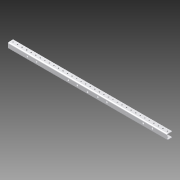
# Autodesk Inventor part: am-0202
Saved by Autodesk Inventor 2012 (Build 160160000, 160)
## iProperties
Category: Chassis
Company: Autodesk Inc.
Created: 2011-12-29
Part Number: am-0202
Document SubType Name: Modeling
Designer: Autodesk Inc.
Density: 1 g/cm^3
Catalog Web Link: http://www.andymark.com/ProductDetails.asp?ProductCode=am%2D0202
Description: C-Channel aluminum piece, for use in the C-Base Drive Chassis.  6 of these items come standard in the C-Base, but only 1 is sh
Vendor: AndyMark
Material: Default
Author: Autodesk Inc.
Autodesk Inventor part; units mm, degrees
ref_plane "YZ Plane" through (0, 0, 0) normal (1, 0, 0) x (0, 1, 0)
ref_plane "XZ Plane" through (0, 0, 0) normal (0, 1, 0) x (-1, 0, 0)
ref_plane "XY Plane" through (0, 0, 0) normal (0, 0, 1) x (1, 0, 0)
sketch "Sketch1" plane through (0, 0, 0) normal (0, 0, 1) x (1, 0, 0)
  line L0 (5.9771, 0) -> (28.2021, 0)
  line L1 (28.2021, 0) -> (28.2021, 3.175)
  line L2 (28.2021, 3.175) -> (5.9771, 3.175)
  line L3 (2.8021, 6.35) -> (2.8021, 25.4)
  line L4 (5.9771, 28.575) -> (28.2021, 28.575)
  line L5 (28.2021, 28.575) -> (28.2021, 31.75)
  line L6 (28.2021, 31.75) -> (5.9771, 31.75)
  line L7 (-0.3729, 25.4) -> (-0.3729, 6.35)
  arc A0 (5.9771, 28.575) -> (2.8021, 25.4) centre (5.9771, 25.4) ccw
  arc A1 (2.8021, 6.35) -> (5.9771, 3.175) centre (5.9771, 6.35) ccw
  arc A2 (5.9771, 31.75) -> (-0.3729, 25.4) centre (5.9771, 25.4) ccw
  arc A3 (-0.3729, 6.35) -> (5.9771, 0) centre (5.9771, 6.35) ccw
  point P0 (0, 0)
  point P1 (-0.3729, 0)
  point P2 (2.8021, 3.175)
  point P3 (2.8021, 28.575)
  dimension "d0" = 28.575
  dimension "d1" = 3.175
  dimension "d2" = 25.4
  dimension "d3" = 25.4
  dimension "d4" = 3.175
  dimension "d5" = 3.175
  dimension "d6" = 6.35
  constraints: 16 end point, 8 point on circle, 8 tangent, 6 point on line, 5 parallel, 4 centre point, 2 equal radius, 1 collinear, 1 horizontal, 1 perpendicular
  measures "d0" distance of point (-0.373, 0) L0.end
  measures "d1" distance of L0.end L1.end
  measures "d2" distance of L1.end point (2.802, 3.175)
  measures "d3" distance of point (2.802, 3.175) point (2.802, 28.575)
  measures "d4" distance of L4.end L5.end
  measures "d5" radius of A0
  measures "d6" radius of A2
extrude "Extrusion1" add sketch "Sketch1" against normal blind 889
sketch "Sketch2" plane through (-0.3729, 6.35, 0) normal (-1, 0, 0) x (0, 0, 1)
  line L0 (0, 19.05) -> (-889, 19.05) projected
  line L1 (-228.6, 0) -> (-228.6, 7.9375)
  arc A0 (-228.6, 11.1125) -> (-228.6, 7.9375) centre (-228.6, 9.525) ccw
  line L2 (-228.6, 11.1125) -> (-228.6, 19.05)
  line L3 (-228.6, 19.05) -> (-889, 19.05)
  line L4 (-889, 0) -> (-889, 19.05)
  line L5 (-889, 0) -> (-228.6, 0)
  circle A1 centre (-552.45, 11.43) radius 4.826
  circle A2 centre (-501.65, 11.43) radius 4.826
  circle A3 centre (-387.35, 11.43) radius 4.826
  circle A4 centre (-336.55, 11.43) radius 4.826
  circle A5 centre (-444.5, 7.62) radius 4.826
  circle A6 centre (-730.25, 11.43) radius 4.826
  circle A7 centre (-781.05, 11.43) radius 4.826
  line L6 (0, 25.4) -> (-889, 25.4) construction
  circle A8 centre (-133.35, 11.43) radius 4.826
  circle A9 centre (-82.55, 11.43) radius 4.826
  point P0 (0, -6.35)
  point P1 (-254, 0.852)
  dimension "d10" = 7.62
  dimension "d11" = 3.81
  dimension "d14" = 254
  constraints: 10 centre point, 10 end point, 2 point on circle, 1 horizontal, 4 other
  measures "d10" distance from line of L0 A7.centre
  measures "d11" vertical distance of A5.centre A7.centre
  measures "d14" distance of A4.centre A9.centre
hole "Hole1" at (-0.3729, 17.78, -781.05) at (-0.3729, 17.78, -730.25) at (-0.3729, 17.78, -552.45) at (-0.3729, 17.78, -501.65) at (-0.3729, 13.97, -444.5) at (-0.3729, 17.78, -387.35) at (-0.3729, 17.78, -336.55) at (-0.3729, 17.78, -133.35) at (-0.3729, 17.78, -82.55) direction (1, 0, 0) diameter 9.652 end through all
hole "Hole2" at (-0.3729, 15.875, -228.6) direction (1, 0, 0) diameter 3.175 end through all
sketch "Sketch3" plane through (5.9771, 31.75, 0) normal (0, 1, 0) x (1, 0, 0)
  line L0 (22.225, 889) -> (0, 889) projected
  line L1 (22.225, 0) -> (22.225, 889) projected
  point P0 (-5.9771, 0)
  point P1 (9.525, 876.3)
  dimension "d34" = 12.7
  dimension "d35" = 12.7
  measures "d34" distance from line of point (9.525, 876.3) L0
  measures "d35" distance from line of point (9.525, 876.3) L1
hole "Hole3" at (15.5021, 31.75, -876.3) direction (0, -1, 0) diameter 6.5278 end through all
pattern_linear "Rectangular Pattern1" count 35 spacing 25.4 along (0, 0, 1) of "Hole3"
equation "\"d35\" = d34"
body "Solid1"
